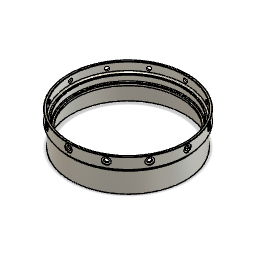
Baugruppe-Segmentverbinder-21.10.2024 v5 (Autodesk Fusion 360 archive; units mm, degrees)
design "Connection-Ring-female-21.10.2024"
Autodesk Fusion 360 part; units mm, degrees
sketch "Skizze1" plane through (0, 0, 0) normal (0, 0, 1) x (1, 0, 0)
  line L0 (-83, 47) -> (-83, 30)
  line L1 (-83, 30) -> (-80, 30)
  line L2 (-80, 30) -> (-80, 0)
  line L3 (-73, 22.5) -> (-73, 25.5)
  line L4 (-73, 25.5) -> (-76, 25.5)
  line L5 (-76, 25.5) -> (-76, 34)
  line L6 (-76, 34) -> (-80, 34)
  line L7 (-80, 34) -> (-80, 47)
  line L8 (-80, 47) -> (-83, 47)
  line L9 (-80, 0) -> (-79, 0)
  line L10 (-76.75, 22.5) -> (-73, 22.5)
  line L11 (-76.75, 22.5) -> (-79, 0)
  line L12 (-76, 30) -> (-76.75, 22.5)
  dimension "d2" = 3
  dimension "d6" = 13
  dimension "d7" = 80
  dimension "d8" = 3
  dimension "d9" = 4
  dimension "d10" = 3
  dimension "d21" = 4
  dimension "d22" = 8.5
  dimension "d23" = 3
  dimension "d24" = 30
  dimension "d25" = 1
  constraint vertical L0
  constraint perpendicular L0 L1
  constraint perpendicular L1 L2
  constraint perpendicular L2 L4
  constraint perpendicular L5 L6
  constraint perpendicular L6 L7
  constraint perpendicular L0 L8
  constraint perpendicular L2 L9
  constraint horizontal origin L2.end
  constraint coincident L5 L12.start
  constraint collinear L11 L12
  constraint horizontal L1.end L12.start
  measures "d2" distance of L3 L5
  measures "d6" distance of L6 L8
  measures "d7" distance of origin L2
  measures "d8" distance of L0 L7
  measures "d9" distance of L2 L5
  measures "d10" distance of L0 L2
  measures "d21" distance of L1 L6
  measures "d22" distance of L4 L6
  measures "d23" distance of L4 L10
  measures "d24" distance of L1 L9
  measures "d25" distance of L2.end L9.end
revolve "Drehen1" add sketch "Skizze1" angle 360 about axis through (0, 1.75, 0) along (0, 1, 0)
fillet "Abrundung1" radius 2 1 edges at (-77.3832, 30, 30.0141)
fillet "Abrundung2" radius 2 1 edges at (-74.5862, 30, 28.9292)
fillet "Abrundung3" radius 2 1 edges at (-74.5862, 34, 28.9292)
chamfer "Fase3" distance 1 angle 45 1 edges at (-70.8569, 25.5, 27.4828)
ref_plane "Arbeitsebene1" through (83, 38.5, 0) normal (1, 0, 0) x (0, 0, -1)
sketch "Skizze4" plane through (83, 0, 0) normal (1, 0, 0) x (0, 0, -1)
  line L0 (-82.5, 47) -> (82.5, 47)
  point P0 (0, 40.5)
  dimension "d34" = 6.5
  constraint vertical origin P0
  measures "d34" distance of P0 L0
hole "Bohrung2" at (83, 40.5, 0) direction (-1, 0, 0) diameter 5.5 depth 16 tip angle 118 counterbore diameter 10 counterbore depth 1
pattern_circular "C-Anordnung1" count 12 over 360 about axis through (0, 1.75, 0) along (0, 1, 0) of "Bohrung2"
chamfer "Fase4" distance 0.4 angle 45 7 edges at (-74.5862, 47, 28.9292) (-70.8569, 34, 27.4828) (-74.5862, 0, 28.9292) (-73.6539, 0, 28.5676) (-71.5561, 22.5, 27.754) (-68.0599, 22.5, 26.3979) (-77.3832, 47, 30.0141)
equation "d7 = ( 160 / 2 ) * 1 mm"
equation "d22 = 15 mm - d6 / 2"

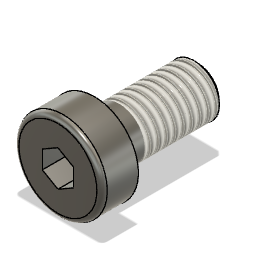
design "Innensechskantschraube DIN 7984 - M5 x 10 Stahl 8.8 Einfach"
description: Innensechskantschraube DIN 7984 - M5 x 10
Autodesk Fusion 360 part; units mm, degrees
sketch "Sketch1" plane through (0, 0, 0) normal (0, 1, 0) x (1, 0, 0)
  line L0 (-2.5, 0) -> (-2.5, 10)
  line L1 (-2.5, 10) -> (0, 10)
  line L2 (0, 10) -> (0, -3.5)
  line L3 (-2.5, 0) -> (-4.25, 0)
  line L4 (-4.25, 0) -> (-4.25, -3.5)
  line L5 (-4.25, -3.5) -> (0, -3.5)
  dimension "d9" = 5
  dimension "d66" = 8.5
  dimension "d68" = 10
  dimension "d79" = 3.5
  constraint perpendicular L0 L1
  constraint collinear origin L1.end L2.end
  constraint perpendicular L0 L3
  constraint coincident origin L3
  constraint vertical L0
  constraint vertical L2
  constraint parallel L2 L4
  constraint coincident L2 L5.end
  constraint perpendicular L2 L5
  measures "d68" distance of origin L1.end
  measures "d79" distance of L3.end L4.end
revolve "Revolve1" add sketch "Sketch1" angle 360 about axis through (0, 0, -10) along (0, 0, 1)
ref_plane "WorkPlane1" through (0, 0, 3.5) normal (0, 0, 1) x (1, 0, 0)
sketch "Sketch6" plane through (0, 0, 3.5) normal (0, 0, 1) x (1, 0, 0)
  line L0 (-1.5, 0) -> (1.5, 0) construction
  line L1 (0, 0) -> (-1.5, 0.866)
  line L2 (-1.5, -0.866) -> (-1.5, 0.866)
  line L3 (-1.5, -0.866) -> (0, 0)
  dimension "d72" = 3
  dimension "d100" = 150
  constraint horizontal L0
  constraint midpoint L1.start L0
  constraint coincident L1.start L3.end
  constraint perpendicular L0 L2
  constraint midpoint L0.start L2
  constraint coincident L1.end L2.end
  measures "d72" distance of L0.start L0.end
  measures "d100" angle of L0 L1
extrude "Extrude1" cut sketch "Sketch6" against normal blind 2.7
pattern_circular "C-Pattern1" count 6 over 360 about axis through (0, 0, 1.75) along (0, 0, 1) of "Extrude1"
extrude "Extrude2" cut 1 faces at (0, -0.5774, 0.8) along direction (0, 0, -1) blind 2.7 draft -85
thread "Thread2" "ISO Metric profile 5.0 M5x0.8 6g" major diameter 4.901 minor diameter 3.9895 pitch 0.8 angle 60 resizes the face on face at (-2.4876, 0.2489, -3.3333) from (0, 0, -2.4) to (0, 0, -10)
fillet "Fillet4" radius 0.5 1 edges at (-3.9624, 1.5369, 3.5)
sketch "Sketch7" plane through (0, 0, 0) normal (0, 1, 0) x (1, 0, 0)
  line L0 (-2.55, 10) -> (-2.55, 9.5092)
  line L1 (-2.55, 9.5092) -> (-2.0092, 10)
  line L2 (0, 10) -> (0, -3.5)
  line L3 (-2.55, 10) -> (0, 10)
  dimension "d92" = 0.4908
  dimension "d98" = 2.0092
  dimension "d99" = 2.55
  constraint coincident L2.start L3.end
  constraint perpendicular L2 L3
  constraint coincident L1.end L3
  constraint perpendicular L0 L3
  measures "d92" vertical distance of L0.end L1.end
  measures "d98" horizontal distance of origin L1.end
  measures "d99" distance of origin L0
revolve "Revolve3" cut sketch "Sketch7" angle 360 about axis through (0, 0, 1.75) along (0, 0, 1)
equation "d9 = adsk_nomdia"
equation "adsk_nomlen = 10.00 mm"
equation "adsk_headh = 3.50 mm"
equation "adsk_headdia = 8.50 mm"
equation "adsk_nomdia = 5.00 mm"
equation "adsk_philwidth = 3.00 mm"
equation "d31 = -adsk_phildepth"
equation "adsk_phildepth = 2.70 mm"
equation "d66 = adsk_headdia"
equation "d68 = adsk_nomlen"
equation "d71 = adsk_headh"
equation "d72 = adsk_philwidth"
equation "d76 = -adsk_phildepth"
equation "d79 = adsk_headh"
equation "adsk_thrlen = 7.60 mm"
equation "d84 = adsk_thrlen"
equation "d86 = adsk_nomdia * 0.1"
equation "d92 = adsk_startlen"
equation "adsk_startlen = 0.49076 mm"
equation "adsk_endpointdia = 4.01848 mm"
equation "d98 = adsk_endpointdia / 2"
equation "d99 = adsk_nomdia * 0.51"

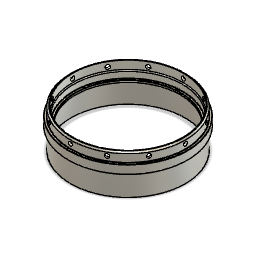
design "Connection-Ring-male-21.10.2024"
Autodesk Fusion 360 part; units mm, degrees
sketch "Skizze1" plane through (0, 0, 0) normal (0, 0, 1) x (1, 0, 0)
  line L0 (-80, 0) -> (-80, 30)
  line L1 (-80, 30) -> (-83, 30)
  line L2 (-83, 30) -> (-83, 42)
  line L3 (-83, 42) -> (-79.95, 42)
  line L4 (-79.95, 42) -> (-79.95, 53)
  line L5 (-77.95, 55) -> (-76.95, 55)
  line L6 (-76.95, 55) -> (-76.95, 42)
  line L7 (-76, 33.5) -> (-73, 33.5)
  line L8 (-73, 30.5) -> (-73, 33.5)
  line L9 (-77.95, 55) -> (-79.95, 53)
  line L10 (-80, 0) -> (-79, 0)
  line L11 (-73, 30.5) -> (-75.95, 30.5)
  line L12 (-75.95, 30.5) -> (-79, 0)
  line L13 (-76, 30) -> (-75.95, 30.5)
  line L14 (-76.95, 42) -> (-76, 42)
  line L15 (-76, 42) -> (-76, 33.5)
  dimension "d1" = 3
  dimension "d2" = 80
  dimension "d5" = 3
  dimension "d7" = 3.05
  dimension "d9" = 2
  dimension "d10" = 3
  dimension "d13" = 1
  dimension "d14" = 30
  dimension "d16" = 2
  dimension "d17" = 4
  dimension "d18" = 8.5
  dimension "d19" = 13
  dimension "d20" = 12
  dimension "d25" = 3
  constraint perpendicular L0 L1
  constraint perpendicular L1 L2
  constraint perpendicular L2 L3
  constraint perpendicular L3 L4
  constraint perpendicular L4 L5
  constraint perpendicular L3 L6
  constraint perpendicular L4 L7
  constraint perpendicular L7 L8
  constraint perpendicular L0 L10
  constraint vertical L8
  constraint perpendicular L8 L11
  constraint horizontal origin L0.start
  constraint collinear L12 L13
  constraint horizontal L0.end L13.start
  constraint perpendicular L6 L14
  constraint perpendicular L14 L15
  constraint vertical L7.start L13.start
  constraint collinear L3 L14
  measures "d1" distance of L7.end L8.start
  measures "d2" distance of origin L0
  measures "d5" distance of L4 L6
  measures "d7" distance of L2 L4
  measures "d9" distance of L4 L5.start
  measures "d10" distance of L0 L2
  measures "d13" distance of L0.start L10.end
  measures "d14" distance of L1 L10
  measures "d16" distance of L5 L4.end
  measures "d17" distance of L0.end L13.start
  measures "d18" distance of L3 L7
  measures "d19" distance of L3 L5
  measures "d20" distance of L1 L3
  measures "d25" distance of L8 L15
revolve "Drehen1" add sketch "Skizze1" angle 360 about axis through (0, 1.75, 0) along (0, 1, 0)
fillet "Abrundung1" radius 2 1 edges at (-71.7426, 42, 27.8263)
ref_plane "Arbeitsebene1" through (79.95, 47.5, 0) normal (1, 0, 0) x (0, 0, -1)
sketch "Skizze2" plane through (79.95, 0, 0) normal (1, 0, 0) x (0, 0, -1)
  line L0 (77.95, 55) -> (-77.95, 55)
  point P0 (0, 48.5)
  dimension "d27" = 6.5
  constraint vertical origin P0
  measures "d27" distance of P0 L0
hole "Bohrung1" at (79.95, 48.5, 0) direction (-1, 0, 0) diameter 5.5 depth 16 tip angle 118
pattern_circular "C-Anordnung1" count 12 over 360 about axis through (0, 1.75, 0) along (0, 1, 0) of "Bohrung1"
chamfer "Fase1" distance 0.4 angle 45 9 edges at (-77.3832, 42, 30.0141) (-77.3832, 30, 30.0141) (-73.6539, 0, 28.5676) (-70.8103, 30.5, 27.4647) (-68.0599, 30.5, 26.3979) (-70.8569, 33.5, 27.4828) (-74.5396, 42, 28.9112) (-74.5862, 0, 28.9292) (-68.0599, 33.5, 26.3979)
fillet "Abrundung2" radius 2 1 edges at (-74.5862, 30, 28.9292)
equation "d2 = ( 160 / 2 ) * 1 mm"
equation "d18 = 15 mm - d19 / 2"
